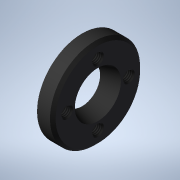
# Autodesk Inventor part: 61581400_2
Saved by Autodesk Inventor 2021 (Build 250183000, 183)
## iProperties
Created: 2026-05-06
Part Number: 61581400_2
Material: Generic
Catalog Web Link: www.3dfindit.com
Description: at_dgb_schrschei_st-Outer part with through hole, Shrink Disks ST, For very high torques
Vendor: MAEDLER
Document SubType Name: Modeling
Designer: psAdmin
Manufacturer: MAEDLER
Mass: 5.51415 g
Surface Area: 30.9133 cm^2
Volume: 5.51415 cm^3
Density: 1 g/cm^3
Appearance: PSOLRGB-176-176-176
Category: PARTsolutions
Company: MAEDLER
Title: 61581400
Author: Cadenas PARTsolutions
Comments: Outer part with through hole, Shrink Disks ST, For very high torques
PSOL_IDENT_0: {$CADENAS_DATA/23d-libs/maedler/antriebselemente/spannbuchsen_und_spannsaetze/schrumpfscheiben/schru
PSOL_IDENT_1: mpfscheibe_st/at_dgb_schrschei_st.prj},171 {VTYP=3D},{NB=61581400_2},{LINA=61581400},{NN=at_dgb_schr
PSOL_IDENT_2: schei_st},{DATE=02.01.2025 14:04:17},{GEOMDATE=02.01.2025 14:04:00},{VERSION=},{LINEID=20},{WBVAR=},
PSOL_IDENT_3: {WBNUMERIC=}  {NB=61581400_2},{LINA=61581400},{KT=DUMMY},{ARTNR=61581400},{WEBSHOP=Produktdetails /
PSOL_IDENT_4: Katalogseite / Montageanleitung},{MATK=Stahl},{MAT=Hochwertiger Stahl 42CrMo4},{ID=14},{DW=10 / 11 /
PSOL_IDENT_5: 12},{DM=40 / 50 / 65},{D=38},{L=15.0},{L2=18.5},{I=10},{E=2.50},{PSMAX=0.014},{SCHR= 4 x M5 x 12},{
PSOL_IDENT_6: TA=3},{PW=154 / 191 / 243},{GEW=0.10},{TK=26.0},{SSA=4},{SSG=5},{SSL=12},{K=3.5},{SDW=6.9},{SW=8},{H
PSOL_IDENT_7: DW=0.5},{DG=5.3},{D1L=20.00},{D2L=16.80},{SL=1.70},{HD=35.6},{BA=6.650},{TN=at_dgb_schrschei_st_14},
PSOL_IDENT_8: {CTN=84839089},{DIST=1.883333}
NB: 61581400_2
NN: at_dgb_schrschei_st
NT: Outer part with through hole, Shrink Disks ST, For very high torques
NBSYN: $ARTNR._2
LINA: 61581400
CATALOG: MÄDLER
ARTNR: 61581400
WEBSHOP: Product details / Catalogue page / Assembly instructions
MATK: Steel
MAT: High-quality steel 42CrMo4
ID: 14
DW: 10 / 11 / 12
DM: 40 / 50 / 65
D: 38
L: 15
L2: 18.5
I: 10
E: 2.5
PSMAX: 0.014
SCHR: 4 x M5 x 12
TA: 3
PW: 154 / 191 / 243
GEW: 0.1
TK: 26
SSA: 4
SSG: 5
SSL: 12
K: 3.5
SDW: 6.9
SW: 8
HDW: 0.5
DG: 5.3
D1L: 20
D2L: 16.8
SL: 1.7
HD: 35.6
BA: 6.65
TN: at_dgb_schrschei_st_14
CTN: 84839089
SUPPLIER: MAEDLER
ARTICLENO: 61581400_2
BOMINFO: 61581400
CREATOR: CADENAS GmbH
Autodesk Inventor part; units mm, degrees
sketch "Sketch_10" plane through (0, 0, 0) normal (0, 0, 1) x (1, 0, 0)
  line L0 (6.65, 0) -> (0, 0)
  line L1 (0, 0) -> (0, 19)
  line L2 (0, 19) -> (5.45, 19)
  line L3 (5.45, 19) -> (6.65, 17.8)
  line L4 (6.65, 17.8) -> (6.65, 0)
  line L5 (6.65, 0) -> (0, 0)
  constraints: 12 end point
revolve "Revolution1" add sketch "Sketch_10" angle 360 about axis through (6.65, 0, 0) along (1, 0, 0)
sketch "Sketch_11" plane through (0, 0, 0) normal (0, 0, 1) x (1, 0, 0)
  line L0 (6.65, 0) -> (0, 0)
  line L1 (0, 0) -> (0, 7.6)
  line L2 (0, 7.6) -> (6.65, 9.728)
  line L3 (6.65, 9.728) -> (6.65, 0)
  line L4 (6.65, 0) -> (0, 0)
  constraints: 10 end point
revolve "Revolution2" cut sketch "Sketch_11" angle 360 about axis through (6.65, 0, 0) along (1, 0, 0)
sketch "Sketch_12" plane through (0, 0, 0) normal (0, 0, 1) x (1, 0, 0)
  line L0 (6.65, 13) -> (0, 13)
  line L1 (0, 13) -> (0, 15.5)
  line L2 (0, 15.5) -> (0.433, 15.067)
  line L3 (0.433, 15.067) -> (6.217, 15.067)
  line L4 (6.217, 15.067) -> (6.65, 15.5)
  line L5 (6.65, 15.5) -> (6.65, 13)
  line L6 (6.65, 13) -> (0, 13)
  constraints: 14 end point
revolve "Revolution3" cut sketch "Sketch_12" angle 360 about axis through (6.65, 13, 0) along (1, 0, 0)
thread "Thread1" size "M5x0.8" class "6H" standard "ISO Metric profile" full length
pattern_linear "Rectangular Pattern1" count 2 spacing 18.3848 along (0, -0.7071, 0.7071) count 2 spacing 18.3848 along (0, -0.7071, -0.7071) of "Revolution3"
ref_plane "at1_dgb_st_XY" through (0, 0, 0) normal (1, 0, 0) x (0, 0, -1)
ref_plane "at1_dgb_st_YZ" through (0, 0, 0) normal (0, 0, -1) x (0, 1, 0)
ref_plane "at1_dgb_st_ZX" through (0, 0, 0) normal (0, 1, 0) x (1, 0, 0)
ref_plane "at_gew_XY" through (15, 0, 0) normal (1, 0, 0) x (0, 0, -1)
ref_plane "at_gew_YZ" through (15, 0, 0) normal (0, 0, -1) x (0, 1, 0)
ref_plane "at_gew_ZX" through (15, 0, 0) normal (0, 1, 0) x (1, 0, 0)
ref_plane "it_schrschei_XY" through (7.5, 0, 0) normal (1, 0, 0) x (0, 0, -1)
ref_plane "it_schrschei_YZ" through (7.5, 0, 0) normal (0, 0, -1) x (0, 1, 0)
ref_plane "it_schrschei_ZX" through (7.5, 0, 0) normal (0, 1, 0) x (1, 0, 0)
body "Solid1"
